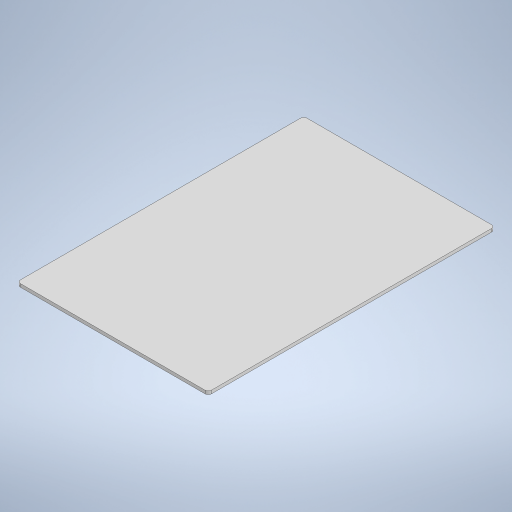
# Autodesk Inventor part: piastra_motore
Saved by Autodesk Inventor 2023 (Build 270158000, 158)
## iProperties
Created: 2022-08-22
Part Number: piastra_motore
Material: Generico
Document SubType Name: Modeling
Designer: matte
Density: 1 g/cm^3
Appearance: Default
Author: matte
Autodesk Inventor part; units mm, degrees
ref_plane "YZ Plane" through (0, 0, 0) normal (1, 0, 0) x (0, 1, 0)
ref_plane "XZ Plane" through (0, 0, 0) normal (0, 1, 0) x (-1, 0, 0)
ref_plane "XY Plane" through (0, 0, 0) normal (0, 0, 1) x (1, 0, 0)
sketch "Schizzo1" plane through (0, 0, 0) normal (0, 1, 0) x (-1, 0, 0)
  line L0 (98.0469, 110.8594) -> (-21.9531, 110.8594)
  line L1 (-21.9531, 110.8594) -> (-21.9531, -69.1406)
  line L2 (-21.9531, -69.1406) -> (98.0469, -69.1406)
  line L3 (98.0469, -69.1406) -> (98.0469, 110.8594)
  point P0 (0, 0)
  dimension "d2" = 120
  dimension "d3" = 180
  constraints: 8 end point, 2 parallel, 1 horizontal, 1 perpendicular
  measures "d2" distance of L1.end L2.end
  measures "d3" distance of L0.end L1.end
extrude "Estrusione1" add sketch "Schizzo1" along normal blind 2
fillet "Raccordo1" radius 2 4 edges at (21.9531, 1, 110.8594) (21.9531, 1, -69.1406) (-98.0469, 1, -69.1406) (-98.0469, 1, 110.8594)
